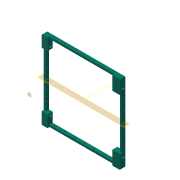
# Autodesk Inventor part: 30_CUBE_openSIM_base_v3
Saved by Autodesk Inventor 2019 (Build 230136000, 136)
## iProperties
Created: 2019-07-01
Part Number: 30_CUBE_openSIM_base_v3
Material: Generic
Document SubType Name: Modeling
Designer: diederichbenedict
Density: 1 g/cm^3
Appearance: IPHT_Türkis
Author: diederichbenedict
Autodesk Inventor part; units mm, degrees
ref_plane "YZ Plane" through (0, 0, 0) normal (1, 0, 0) x (0, 1, 0)
ref_plane "XZ Plane" through (0, 0, 0) normal (0, 1, 0) x (-1, 0, 0)
ref_plane "XY Plane" through (0, 0, 0) normal (0, 0, 1) x (1, 0, 0)
ref_plane "Work Plane1" through (181.6, 41.8, 16) normal (0, 0, -1) x (-1, 0, 0)
sketch "Sketch1" plane through (181.6, 41.8, 16) normal (0, 0, -1) x (-1, 0, 0)
  circle A0 centre (0.9, -0.9) radius 1.45 construction
  line L0 (4, -1.5) -> (1.5, -4) construction
  line L1 (4, -1.5) -> (4, 4) construction
  line L2 (4, 4) -> (-2, 4) construction
  arc A1 (-2, 4) -> (-4, 2) centre (-2, 2) ccw construction
  line L3 (-4, 2) -> (-4, -4) construction
  line L4 (-4, -4) -> (1.5, -4) construction
  arc A2 (45.8, 2) -> (43.8, 4) centre (43.8, 2) ccw construction
  line L5 (43.8, 4) -> (37.8, 4) construction
  line L6 (37.8, 4) -> (37.8, -1.5) construction
  line L7 (40.3, -4) -> (45.8, -4) construction
  line L8 (45.8, -4) -> (45.8, 2) construction
  circle A3 centre (40.9, -0.9) radius 1.45 construction
  line L9 (37.8, -40.3) -> (40.3, -37.8) construction
  line L10 (37.8, -40.3) -> (37.8, -45.8) construction
  line L11 (37.8, -45.8) -> (43.8, -45.8) construction
  arc A4 (43.8, -45.8) -> (45.8, -43.8) centre (43.8, -43.8) ccw construction
  line L12 (45.8, -43.8) -> (45.8, -37.8) construction
  line L13 (45.8, -37.8) -> (40.3, -37.8) construction
  circle A5 centre (40.9, -40.9) radius 1.45 construction
  circle A6 centre (0.9, -40.9) radius 1.45 construction
  line L14 (1.5, -37.8) -> (4, -40.3) construction
  line L15 (1.5, -37.8) -> (-4, -37.8) construction
  line L16 (-4, -37.8) -> (-4, -43.8) construction
  arc A7 (-4, -43.8) -> (-2, -45.8) centre (-2, -43.8) ccw construction
  line L17 (-2, -45.8) -> (4, -45.8) construction
  line L18 (4, -45.8) -> (4, -40.3) construction
  line L19 (40.3, -4) -> (37.8, -1.5) construction
  line L20 (-52, 154) -> (143.8, 154)
  line L21 (145.8, 152) -> (145.8, -43.8)
  line L22 (143.8, -45.8) -> (-52, -45.8)
  line L23 (-54, -43.8) -> (-54, 152)
  line L24 (140.3, -37.8) -> (140.3, 146)
  line L25 (137.8, 148.5) -> (-46, 148.5)
  line L26 (-48.5, 146) -> (-48.5, -37.8)
  line L27 (-46, -40.3) -> (137.8, -40.3)
  line L28 (137.8, -40.3) -> (140.3, -37.8)
  line L29 (-46, -40.3) -> (-48.5, -37.8)
  line L30 (-46, 148.5) -> (-48.5, 146)
  line L31 (140.3, 146) -> (137.8, 148.5)
  arc A8 (145.8, 152) -> (143.8, 154) centre (143.8, 152) ccw
  arc A9 (143.8, -45.8) -> (145.8, -43.8) centre (143.8, -43.8) ccw
  arc A10 (-54, -43.8) -> (-52, -45.8) centre (-52, -43.8) ccw
  arc A11 (-52, 154) -> (-54, 152) centre (-52, 152) ccw
  circle A12 centre (140.8, -40.8) radius 1.4
  circle A13 centre (-49, -40.8) radius 1.4
  circle A14 centre (45.9, 54.1) radius 94.4 construction
  line L32 (45.9, 148.5) -> (45.9, -40.3)
  line L33 (77.4, 111.7) -> (64.2, 111.7) construction
  line L34 (64.2, 96.7) -> (77.4, 96.7) construction
  line L35 (77.4, 61.7) -> (64.2, 61.7) construction
  line L36 (64.2, 46.7) -> (77.4, 46.7) construction
  circle A15 centre (140.8, 149) radius 1.4
  circle A16 centre (-49, 149) radius 1.4
  point P0 (145.8, -45.8)
  point P1 (145.8, 154)
  point P2 (-54, -45.8)
  point P3 (140.3, -40.3)
  point P4 (140.3, 148.5)
  point P5 (-48.5, 148.5)
  point P6 (-48.5, -40.3)
  point P7 (40.8, 149)
  point P8 (45.8, -40.8)
  point P9 (70.9, 96)
  dimension "d34" = 199.8
  dimension "d35" = 199.8
  dimension "d36" = 5.5
  dimension "d37" = 2.5
  dimension "d38" = 2.5
  dimension "d39" = 2.5
  dimension "d40" = 2.5
  dimension "d41" = 2.5
  dimension "d42" = 2.5
  dimension "d43" = 2.5
  dimension "d44" = 2.5
  dimension "d45" = 2
  dimension "d46" = 5
  dimension "d47" = 5
  dimension "d48" = 5
  dimension "d49" = 5
  dimension "d51" = 5
  dimension "d57" = 2.8
  dimension "d58" = 2.8
  dimension "d255" = 2.8
  dimension "d256" = 5
  dimension "d257" = 5
  dimension "d308" = 2.8
  dimension "d309" = 5
  dimension "d310" = 5
  constraints: 26 end point, 14 point on line, 8 centre point, 8 point on circle, 8 tangent, 7 coincident, 4 parallel, 3 equal radius, 3 midpoint, 2 horizontal, 2 perpendicular, 2 vertical, 1 vertical alignment, 5 other
  measures "d34" distance of point (145.8, -45.8) point (-54, -45.8)
  measures "d35" distance of point (145.8, 154) point (145.8, -45.8)
  measures "d36" distance between parallel lines of L21 L24
  measures "d37" distance of L27.end point (140.3, -40.3)
  measures "d38" distance of L24.start point (140.3, -40.3)
  measures "d39" distance of L27.start point (-48.5, -40.3)
  measures "d40" distance of L26.end point (-48.5, -40.3)
  measures "d41" distance of L25.end point (-48.5, 148.5)
  measures "d42" distance of L26.start point (-48.5, 148.5)
  measures "d43" distance of L24.end point (140.3, 148.5)
  measures "d44" distance of L25.start point (140.3, 148.5)
  measures "d45" radius of A8
  measures "d46" distance from line of point (-49, -40.8) L23
  measures "d47" distance from line of L22 point (-49, -40.8)
  measures "d48" distance from line of L21 point (140.8, -40.8)
  measures "d49" distance from line of L22 point (140.8, -40.8)
  measures "d51" distance from line of L20 point (40.8, 149)
  measures "d57" diameter of A12
  measures "d58" diameter of A13
  measures "d255" diameter of A15
  measures "d256" distance from line of A15.centre L20
  measures "d257" distance from line of A15.centre L21
  measures "d308" diameter of A16
  measures "d309" distance from line of A16.centre L23
  measures "d310" distance from line of A16.centre L20
extrude "Extrusion1" add sketch "Sketch1" along normal blind 8
sketch "Sketch56" plane through (181.6, 41.8, 8) normal (0, 0, -1) x (-1, 0, 0)
  line L0 (137.8, 148.5) -> (140.3, 146) projected
  line L1 (140.3, 146) -> (140.3, -37.8) construction
  line L2 (140.3, -37.8) -> (137.8, -40.3) projected
  line L3 (137.8, -40.3) -> (-46, -40.3) projected
  line L4 (-46, -40.3) -> (-48.5, -37.8) projected
  line L5 (-48.5, -37.8) -> (-48.5, 146) projected
  line L6 (-48.5, 146) -> (-46, 148.5) projected
  line L7 (-46, 148.5) -> (137.8, 148.5) projected
  line L8 (145.8, 152) -> (145.8, -43.8) projected
  arc A0 (143.8, -45.8) -> (145.8, -43.8) centre (143.8, -43.8) ccw projected
  line L9 (143.8, -45.8) -> (-52, -45.8) projected
  arc A1 (-54, -43.8) -> (-52, -45.8) centre (-52, -43.8) ccw projected
  line L10 (-54, -43.8) -> (-54, 152) projected
  arc A2 (-52, 154) -> (-54, 152) centre (-52, 152) ccw projected
  line L11 (-52, 154) -> (143.8, 154) projected
  arc A3 (145.8, 152) -> (143.8, 154) centre (143.8, 152) ccw projected
  circle A4 centre (140.8, -40.8) radius 1.4 projected
  circle A5 centre (-49, -40.8) radius 1.4 projected
  circle A6 centre (140.8, 149) radius 1.4 projected
  circle A7 centre (-49, 149) radius 1.4 projected
  line L12 (137.8, 148.5) -> (-46, 148.5) projected
  line L13 (-46, 148.5) -> (-48.5, 146) projected
  line L14 (-48.5, 146) -> (-48.5, -37.8) projected
  line L15 (-48.5, -37.8) -> (-46, -40.3) projected
  line L16 (-46, -40.3) -> (137.8, -40.3) projected
  line L17 (137.8, -40.3) -> (140.3, -37.8) projected
  line L18 (140.3, -37.8) -> (140.3, 146) projected
  line L19 (140.3, 146) -> (137.8, 148.5) projected
  line L20 (145.8, -45.8) -> (125.8, -45.8) construction
  line L21 (125.8, -45.8) -> (125.8, -15.8) construction
  line L22 (125.8, -15.8) -> (145.8, -15.8) construction
  line L23 (145.8, -15.8) -> (145.8, -45.8) construction
  line L24 (-54, -45.8) -> (-34, -45.8) construction
  line L25 (-34, -45.8) -> (-34, -10.8) construction
  line L26 (-34, -10.8) -> (-54, -10.8) construction
  line L27 (-54, -10.8) -> (-54, -45.8) construction
  line L28 (145.8, -15.8) -> (130.8, -15.8)
  line L29 (130.8, -15.8) -> (130.8, -45.8)
  line L30 (-54, -10.8) -> (-34, -10.8)
  line L31 (-34, -45.8) -> (-34, -10.8)
  line L32 (145.8, -15.8) -> (145.8, -43.8)
  line L33 (143.8, -45.8) -> (130.8, -45.8)
  line L34 (-54, -10.8) -> (-54, -43.8)
  line L35 (-34, -45.8) -> (-52, -45.8)
  point P0 (181.6, -41.8)
  dimension "d373" = 20
  dimension "d374" = 30
  dimension "d375" = 20
  dimension "d376" = 35
  dimension "d377" = 15
  constraints: 32 end point, 5 point on line, 4 parallel, 3 collinear, 3 perpendicular, 3 point on circle, 2 horizontal, 1 tangent
  measures "d373" distance of L21.end L22.end
  measures "d374" distance of L20.end L21.end
  measures "d375" distance of L26.end L25.end
  measures "d376" distance of L25.end L24.end
  measures "d377" distance of L22.end L28.end
extrude "Extrusion35" add sketch "Sketch56" against normal blind 13 contours L28 L8 A0 L9 L29 L3 L2 L18 | L18 L2 L3 L29 L28 | L30 L31 L3 L4 L5 | L5 L4 L3 L31 L9 A1 L10 L30
sketch "Sketch57" plane through (235.6, -2, 16) normal (1, 0, 0) x (0, 0, -1)
  circle A0 centre (3, 22) radius 3.05
  line L0 (8, 195.8) -> (8, 0) projected
  line L1 (0, 195.8) -> (8, 195.8) projected
  line L2 (0, 33) -> (0, 195.8) projected
  line L3 (0, 33) -> (-5, 33) projected
  line L4 (-5, 0) -> (-5, 33) projected
  line L5 (8, 0) -> (-5, 0) projected
  line L6 (8, -2) -> (-5, -2) projected
  point P0 (16, 2)
  dimension "d379" = 5
  dimension "d380" = 24
  constraints: 1 centre point
  measures "d379" distance from line of A0.centre L0
  measures "d380" distance from line of A0.centre L6
extrude "Extrusion36" cut sketch "Sketch57" against normal through all contours A0
sketch "Sketch59" plane through (181.6, 41.8, 21) normal (0, 0, 1) x (1, 0, 0)
  circle A0 centre (40, -27.1) radius 3.5
  line L0 (54, -43.8) -> (54, -10.8) projected
  line L1 (-170.0796, -30.6) -> (49.9204, -30.6) construction
  line L2 (-170.0796, -30.6) -> (49.9204, -30.6) construction
  arc A1 (-171.5, -32.6) -> (-168.5, -32.6) centre (-170, -34.6) ccw
  circle A2 centre (-170, -34.6) radius 4
  circle A3 centre (48, -35.1) radius 3.5
  line L3 (-170, -38.6) -> (63.6932, -38.6) construction
  line L4 (-170, -38.6) -> (63.6932, -38.6) construction
  point P0 (-181.6, -41.8)
  dimension "d385" = 8
  dimension "d378" = 7
  dimension "d381" = 14
  dimension "d383" = 220
  dimension "d384" = 0
  dimension "d386" = 4
  dimension "d387" = 7
  dimension "d388" = 8
  dimension "d389" = 8
  dimension "d397" = 0
  constraints: 8 end point, 3 centre point, 3 horizontal, 2 collinear, 2 point on circle, 1 coincident, 1 tangent, 1 vertical alignment, 6 other
  measures "d378" diameter of A0
  measures "d381" distance from line of A0.centre L0
  measures "d383" distance of L1.start L1.end
  measures "d384" distance between parallel lines of L1 L2
  measures "d386" distance from line of L1 A1.centre
  measures "d387" diameter of A3
  measures "d388" horizontal distance of A0.centre A3.centre
  measures "d389" horizontal distance of A0.centre A3.centre
  measures "d397" distance between parallel lines of L3 L4
hole "Hole12" at (229.6, 6.7, 21) at (221.6, 14.7, 21) direction (0, 0, -1) diameter 2.9 end through all
sketch "Sketch60" plane through (37.8, -4, 16) normal (0, 1, 0) x (1, 0, 0)
  line L0 (6, 0) -> (189.8, 0) projected
  line L1 (6, 0) -> (6, 8) projected
  line L2 (189.8, 8) -> (6, 8) projected
  line L3 (189.8, 0) -> (189.8, 8) projected
  circle A0 centre (172.8, 4) radius 1.45
  circle A1 centre (43.1531, 4) radius 1.45
  line L4 (197.8, 0) -> (197.8, 8) projected
  circle A2 centre (147.8, 4) radius 1.45
  circle A3 centre (122.8, 4) radius 1.45
  circle A4 centre (97.8, 4) radius 1.45
  circle A5 centre (72.8, 4) radius 1.45
  circle A6 centre (47.8, 4) radius 1.45
  circle A7 centre (22.8, 4) radius 1.45
  point P0 (-37.8, 16)
  dimension "d398" = 2.9
  dimension "d399" = 2.9
  dimension "d400" = 25
  dimension "d401" = 4
  dimension "d404" = 25
  constraints: 8 centre point, 1 horizontal, 12 other
  measures "d398" diameter of A0
  measures "d399" diameter of A1
  measures "d400" distance from line of A0.centre L4
  measures "d401" distance from line of A0.centre L0
  measures "d404" distance of A0.centre A2.centre
hole "Hole13" at (210.6, -4, 12) at (185.6, -4, 12) at (160.6, -4, 12) at (135.6, -4, 12) at (110.6, -4, 12) at (85.6, -4, 12) at (60.6, -4, 12) direction (0, 1, 0) diameter 2.9 end through all
sketch "Sketch61" plane through (235.6, -2, 8) normal (1, 0, 0) x (0, 0, -1)
  line L0 (0, 195.8) -> (0, 0) projected
  line L1 (0, 33) -> (-8, 33) projected
  line L2 (-8, 189.8) -> (-8, 33) projected
  line L3 (-8, 189.8) -> (0, 189.8) projected
  line L4 (0, 33) -> (0, 189.8) projected
  circle A0 centre (-4, 172.8) radius 1.45
  line L5 (-8, 197.8) -> (0, 197.8) projected
  circle A1 centre (-4, 147.8) radius 1.45
  circle A2 centre (-4, 122.8) radius 1.45
  circle A3 centre (-4, 97.8) radius 1.45
  circle A4 centre (-4, 72.8) radius 1.45
  circle A5 centre (-4, 47.8) radius 1.45
  point P0 (8, 2)
  dimension "d416" = 2.9
  dimension "d417" = 25
  dimension "d420" = 25
  constraints: 6 centre point, 1 vertical, 10 other
  measures "d416" diameter of A0
  measures "d417" distance from line of A0.centre L5
  measures "d420" distance of A0.centre A1.centre
hole "Hole14" at (235.6, 45.8, 12) at (235.6, 70.8, 12) at (235.6, 95.8, 12) at (235.6, 120.8, 12) at (235.6, 145.8, 12) at (235.6, 170.8, 12) direction (-1, 0, 0) diameter 2.9 end through all
ref_plane "Work Plane15" through (50.8, 95.9, 16) normal (0, 1, 0) x (1, 0, 0)
mirror "Mirror3" about plane through (50.8, 95.9, 16) normal (0, 1, 0) of "Extrusion35", "Extrusion36", "Hole12"
equation "\"d38\" = d37"
equation "\"d39\" = d37"
equation "\"d40\" = d39"
equation "\"d41\" = d37"
equation "\"d42\" = d41"
equation "\"d43\" = d37"
equation "\"d44\" = d43"
body "Solid1"
